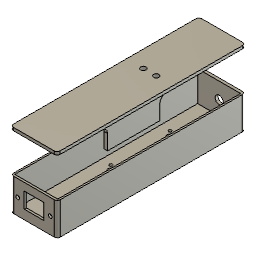
box_bridge_RS485_CAN v7 (Autodesk Fusion 360 design; units mm, degrees)
Autodesk Fusion 360 part; units mm, degrees
sketch "Sketch1" plane through (0, 0, 0) normal (0, 1, 0) x (1, 0, 0)
  line L0 (-27.5618, 41.4437) -> (-7.0618, 41.4437)
  line L1 (-7.0618, 41.4437) -> (-7.0618, -44.5563)
  line L2 (-7.0618, -44.5563) -> (-27.5618, -44.5563)
  line L3 (-27.5618, -44.5563) -> (-27.5618, 41.4437)
  line L4 (-17.3118, 41.4437) -> (-17.3118, -44.5563) construction
  line L5 (-7.0618, -1.5563) -> (-27.5618, -1.5563) construction
  line L6 (-7.0618, 24.2704) -> (-27.5618, 24.2704) construction
  line L7 (-17.3118, 24.2704) -> (-17.3118, -26.7296) construction
  circle A0 centre (-17.3118, 24.2704) radius 1.5
  circle A1 centre (-17.3118, -26.7296) radius 1.5
  dimension "d1" = 20.5
  dimension "d2" = 86
  dimension "d3" = 51
  dimension "d4" = 3
  dimension "d5" = 3
  constraint horizontal L0
  constraint vertical L1
  constraint horizontal L2
  constraint vertical L3
  constraint midpoint L0 L4.start
  constraint midpoint L2 L4.end
  constraint midpoint L1 L5.start
  constraint midpoint L3 L5.end
  constraint coincident L1 L6.start
  constraint coincident L3 L6.end
  constraint perpendicular L3 L6
  constraint midpoint L6 L7.start
  constraint perpendicular L6 L7
  constraint coincident L7.start A0.centre
  constraint coincident L7.end A1.centre
  measures "d1" distance of L0.start L0.end
  measures "d2" distance of L0.end L1.end
  measures "d3" distance of L7.start L7.end
  measures "d4" diameter of A0
  measures "d5" diameter of A1
extrude "Extrude1" add sketch "Sketch1" along normal blind 19.7 makes body 1
sketch "Sketch2" plane through (0, 19.7, 0) normal (0, 1, 0) x (-1, 0, 0)
  circle A0 centre (17.3118, -24.2704) radius 1.5
  circle A1 centre (17.3118, 26.7296) radius 1.5
  line L0 (27.5618, 44.5563) -> (7.0618, 44.5563)
  line L1 (7.0618, 44.5563) -> (7.0618, -41.4437)
  line L2 (7.0618, -41.4437) -> (27.5618, -41.4437)
  line L3 (27.5618, -41.4437) -> (27.5618, 44.5563)
extrude "Extrude2" cut sketch "Sketch2" against normal blind 5 bodies 1
sketch "Sketch3" plane through (0, 14.7, 0) normal (0, 1, 0) x (-1, 0, 0)
  circle A0 centre (17.3118, 26.7296) radius 1.5
  circle A1 centre (17.3118, -24.2704) radius 1.5
  line L0 (27.5618, -41.4437) -> (27.5618, 44.5563)
  line L1 (27.5618, 44.5563) -> (7.0618, 44.5563)
  line L2 (7.0618, 44.5563) -> (7.0618, -41.4437)
  line L3 (7.0618, -41.4437) -> (27.5618, -41.4437)
  line L4 (17.3118, 26.7296) -> (17.3118, 10.2296) construction
  line L5 (17.3118, 10.2296) -> (11.8118, 10.2296) construction
  line L6 (17.3118, 10.2296) -> (22.8118, 10.2296) construction
  circle A2 centre (22.8118, 10.2296) radius 1.75
  circle A3 centre (17.3118, 10.2296) radius 1.75
  circle A4 centre (11.8118, 10.2296) radius 1.75
  dimension "d10" = 16.5
  dimension "d11" = 5.5
  dimension "d12" = 5.5
  dimension "d13" = 3.5
  dimension "d14" = 3.5
  dimension "d15" = 3.5
  constraint coincident A0.centre L4.start
  constraint parallel L2 L4
  constraint perpendicular L4 L5
  constraint perpendicular L4 L6
  constraint coincident L6.end A2.centre
  constraint coincident L4.end L5.start
  constraint coincident L5.end A4.centre
  measures "d10" distance of A0.centre L4.end
  measures "d11" distance of L4.end L5.end
  measures "d12" distance of L4.end L6.end
  measures "d13" diameter of A2
  measures "d14" diameter of A3
  measures "d15" diameter of A4
extrude "Extrude3" add sketch "Sketch3" along normal blind 5 contours A2 | A3 | A4 bodies 1
sketch "Sketch4" plane through (0, 0, 0) normal (0, 0, 1) x (1, 0, 0)
  line L0 (0, 0) -> (40, 0)
  line L1 (40, 0) -> (40, 26)
  line L2 (40, 26) -> (0, 26)
  line L3 (0, 26) -> (0, 0)
  line L4 (0, 0) -> (40, 0) construction
  line L5 (40, 0) -> (40, 6) construction
  line L6 (40, 6) -> (0, 6) construction
  line L7 (0, 6) -> (0, 0) construction
  line L8 (20, 6) -> (20, 26) construction
  line L9 (20, 6) -> (28.5, 6) construction
  line L10 (28.5, 6) -> (28.5, 19.5) construction
  line L11 (28.5, 19.5) -> (20, 19.5) construction
  line L12 (20, 19.5) -> (20, 6) construction
  line L13 (20, 6) -> (11.5, 6) construction
  line L14 (11.5, 6) -> (11.5, 19.5) construction
  line L15 (11.5, 19.5) -> (20, 19.5) construction
  line L16 (20, 19.5) -> (20, 6) construction
  line L17 (0, 0) -> (40, 0) construction
  line L18 (40, 0) -> (40, 12) construction
  line L19 (40, 12) -> (0, 12) construction
  line L20 (0, 12) -> (0, 0) construction
  line L21 (59.0811, 36.4997) -> (20, 36.4997) construction
  line L22 (20, 36.4997) -> (20, 6) construction
  line L23 (20, 6) -> (59.0811, 6) construction
  line L24 (59.0811, 6) -> (59.0811, 36.4997) construction
  line L25 (20, 6) -> (34, 6) construction
  line L26 (34, 6) -> (34, 26) construction
  line L27 (34, 26) -> (20, 26) construction
  line L28 (20, 26) -> (20, 6) construction
  line L29 (20, 6) -> (6, 6) construction
  line L30 (6, 6) -> (6, 26) construction
  line L31 (6, 26) -> (20, 26) construction
  line L32 (20, 26) -> (20, 6) construction
  line L33 (11.5, 6) -> (28.5, 6)
  line L34 (28.5, 6) -> (28.5, 19.5)
  line L35 (28.5, 19.5) -> (11.5, 19.5)
  line L36 (11.5, 19.5) -> (11.5, 6)
  circle A0 centre (34, 12) radius 1.6
  circle A1 centre (6, 12) radius 1.6
  dimension "d18" = 40
  dimension "d19" = 26
  dimension "d20" = 6
  dimension "d21" = 8.5
  dimension "d22" = 13.5
  dimension "d23" = 8.5
  dimension "d24" = 12
  dimension "d25" = 14
  dimension "d26" = 14
  dimension "d27" = 3.2
  dimension "d28" = 3.2
  constraint horizontal L0
  constraint vertical L1
  constraint horizontal L2
  constraint vertical L3
  constraint coincident L0.start L3.end
  constraint horizontal L4
  constraint vertical L5
  constraint horizontal L6
  constraint vertical L7
  constraint midpoint L6 L8.start
  constraint midpoint L2 L8.end
  constraint perpendicular L2 L8
  constraint horizontal L9
  constraint vertical L10
  constraint horizontal L11
  constraint vertical L12
  constraint horizontal L13
  constraint vertical L14
  constraint horizontal L15
  constraint vertical L16
  constraint horizontal L17
  constraint vertical L18
  constraint horizontal L19
  constraint vertical L20
  constraint coincident L1 L18.end
  constraint horizontal L21
  constraint vertical L22
  constraint horizontal L23
  constraint vertical L24
  constraint horizontal L25
  constraint vertical L26
  constraint horizontal L27
  constraint vertical L28
  constraint horizontal L29
  constraint vertical L30
  constraint horizontal L31
  constraint vertical L32
  constraint horizontal L33
  constraint vertical L34
  constraint horizontal L35
  constraint vertical L36
  constraint coincident L19 A0.centre
  constraint coincident L26 A0.centre
  constraint coincident L19 A1.centre
  constraint coincident L30 A1.centre
  measures "d18" distance of L0.start L0.end
  measures "d19" distance of L0.start L2.end
  measures "d20" distance of L0.start L6.end
  measures "d21" distance of L8.start L9.end
  measures "d22" distance of L8.start L11.end
  measures "d23" distance of L8.start L13.end
  measures "d24" distance of L0.start L19.end
  measures "d25" distance of L8.start L25.end
  measures "d26" distance of L8.start L29.end
  measures "d27" diameter of A0
  measures "d28" diameter of A1
extrude "Extrude4" add sketch "Sketch4" along normal blind 1.9 separate body makes body 2
extrude "Extrude5" add 1 faces at (13.3333, 0, 0.6333) along direction (0, -1, 0) blind 2 on bodies 2 bodies 2
sketch "Sketch5" plane through (0, 0, 0) normal (0, 0, -1) x (-1, 0, 0)
  line L0 (-11.5, 19.5) -> (-11.5, 6)
  line L1 (-11.5, 6) -> (-28.5, 6)
  line L2 (-28.5, 6) -> (-28.5, 19.5)
  line L3 (-28.5, 19.5) -> (-11.5, 19.5)
  circle A0 centre (-34, 12) radius 1.6
  circle A1 centre (-6, 12) radius 1.6
  line L4 (0, -2) -> (0, 26)
  line L5 (0, 26) -> (-40, 26)
  line L6 (-40, 26) -> (-40, -2)
  line L7 (-40, -2) -> (0, -2)
  line L8 (-40, -2) -> (0, -2)
  line L9 (0, -2) -> (0, 0)
  line L10 (0, 0) -> (-40, 0)
  line L11 (-40, 0) -> (-40, -2)
  dimension "d33" = 2
  constraint horizontal L8
  constraint vertical L9
  constraint horizontal L10
  constraint vertical L11
  constraint coincident L6.end L7.start
  measures "d33" distance of L6.end L10.end
extrude "Extrude6" add sketch "Sketch5" along normal blind 160 contours L4 L6 L7 L8 L9 L10 L11 bodies 2
sketch "Sketch6" plane through (0, 0, 0) normal (0, 1, 0) x (-1, 0, 0)
  line L0 (0, 0) -> (-40, 0)
  line L1 (-40, 0) -> (-40, -160)
  line L2 (-40, -160) -> (0, -160)
  line L3 (0, -160) -> (0, 0)
  line L4 (-40, -160) -> (0, -160)
  line L5 (0, -160) -> (0, -157.5)
  line L6 (0, -157.5) -> (-40, -157.5)
  line L7 (-40, -157.5) -> (-40, -160)
  dimension "d36" = 2.5
  constraint horizontal L4
  constraint vertical L5
  constraint horizontal L6
  constraint vertical L7
  constraint coincident L1.end L2.start
  measures "d36" distance of L1.end L6.end
extrude "Extrude7" add sketch "Sketch6" along normal blind 26 contours L1 L2 L3 L4 L5 L6 L7 bodies 2
sketch "Sketch7" plane through (0, 0, -160) normal (0, 0, -1) x (-1, 0, 0)
  line L0 (-40, 26) -> (-40, -2)
  line L1 (-40, -2) -> (0, -2)
  line L2 (0, -2) -> (0, 26)
  line L3 (0, 26) -> (-40, 26)
  line L4 (-20, 26) -> (-20, -2) construction
  line L5 (0, 12) -> (-40, 12) construction
  circle A0 centre (-20, 12) radius 3.5
  dimension "d39" = 7
  constraint midpoint L3 L4.start
  constraint midpoint L1 L4.end
  constraint midpoint L2 L5.start
  constraint midpoint L0 L5.end
  constraint midpoint L4 A0.centre
  measures "d39" diameter of A0
extrude "Extrude8" cut sketch "Sketch7" against normal blind 3 contours A0 bodies 2
move_body "Move1" bodies 1 to x (1, 0, 0) y (0, 1, 0) z (0, 0, 1) at (37.1076, 0, -91.1851)
sketch "Sketch8" plane through (0, 0, 0) normal (0, 1, 0) x (-1, 0, 0)
  line L0 (-40, -157.5) -> (0, -157.5)
  line L1 (0, -157.5) -> (0, 0)
  line L2 (0, 0) -> (-40, 0)
  line L3 (-40, 0) -> (-40, -157.5)
  line L4 (-40, -64.3303) -> (0, -64.3303) construction
  line L5 (0, -64.3303) -> (0, -115.3303) construction
  line L6 (0, -115.3303) -> (-40, -115.3303) construction
  line L7 (-40, -115.3303) -> (-40, -64.3303) construction
  line L8 (-20, 0) -> (-20, -157.5) construction
  circle A0 centre (-20, -64.3303) radius 2.5
  circle A1 centre (-20, -115.3303) radius 2.5
  dimension "d42" = 51
  dimension "d43" = 5
  dimension "d44" = 5
  constraint horizontal L4
  constraint vertical L5
  constraint horizontal L6
  constraint vertical L7
  constraint coincident L1 L5.end
  constraint coincident L3 L4.start
  constraint midpoint L2 L8.start
  constraint midpoint L0 L8.end
  constraint midpoint L4 A0.centre
  constraint midpoint L6 A1.centre
  measures "d42" distance of L4.start L6.end
  measures "d43" diameter of A0
  measures "d44" diameter of A1
extrude "Extrude9" add sketch "Sketch8" along normal blind 6 contours A0 | A1 bodies 2
sketch "Sketch9" plane through (0, 6, 0) normal (0, 1, 0) x (-1, 0, 0)
  circle A0 centre (-20, -64.3303) radius 2.5
  circle A1 centre (-20, -64.3303) radius 1.25
  dimension "d47" = -1.25
sketch "Sketch10" plane through (0, 6, 0) normal (0, 1, 0) x (-1, 0, 0)
  circle A0 centre (-20, -115.3303) radius 2.5
  circle A1 centre (-20, -115.3303) radius 1.25
  dimension "d48" = -1.25
extrude "Extrude10" add sketch "Sketch10" along normal blind 4 contours A1 bodies 2
extrude "Extrude11" add sketch "Sketch9" along normal blind 4 contours A1 bodies 2
sketch "Sketch11" plane through (0, 0, 0) normal (0, 1, 0) x (-1, 0, 0)
  circle A0 centre (-20, -64.3303) radius 2.5
  circle A1 centre (-20, -115.3303) radius 2.5
  line L0 (-40, -157.5) -> (0, -157.5)
  line L1 (0, -157.5) -> (0, 0)
  line L2 (0, 0) -> (-40, 0)
  line L3 (-40, 0) -> (-40, -157.5)
  line L4 (-40, 0) -> (-38.5, 0)
  line L5 (-38.5, 0) -> (-38.5, -157.5)
  line L6 (-38.5, -157.5) -> (-40, -157.5)
  line L7 (-40, -157.5) -> (-40, 0)
  line L8 (0, 0) -> (-1.5, 0)
  line L9 (-1.5, 0) -> (-1.5, -157.5)
  line L10 (-1.5, -157.5) -> (0, -157.5)
  line L11 (0, -157.5) -> (0, 0)
  dimension "d53" = 1.5
  dimension "d54" = 1.5
  constraint horizontal L4
  constraint vertical L5
  constraint horizontal L6
  constraint vertical L7
  constraint coincident L2.end L3.start
  constraint horizontal L8
  constraint vertical L9
  constraint horizontal L10
  constraint vertical L11
  constraint coincident L1.end L2.start
  measures "d53" distance of L2.end L4.end
  measures "d54" distance of L1.end L8.end
extrude "Extrude12" add sketch "Sketch11" along normal blind 26 contours L0 L2 L3 L4 L5 L6 L7 | L0 L1 L2 L8 L9 L10 L11 bodies 2
fillet "Fillet1" radius 2.5 4 edges at (0, 12, -160) (0, 12, 1.9) (40, 12, -160) (40, 12, 1.9) on bodies 2
sketch "Sketch12" plane through (0, 0, 0) normal (0, 1, 0) x (-1, 0, 0)
  circle A0 centre (-20, -115.3303) radius 2.5
  circle A1 centre (-20, -64.3303) radius 2.5
  line L0 (-38.5, 0) -> (-38.5, -157.5)
  line L1 (-38.5, -157.5) -> (-1.5, -157.5)
  line L2 (-1.5, -157.5) -> (-1.5, 0)
  line L3 (-1.5, 0) -> (-38.5, 0)
  line L4 (-20, -112.8303) -> (-1.5, -112.8303) construction
  line L5 (-1.5, -112.8303) -> (-1.5, -97.8303) construction
  line L6 (-1.5, -97.8303) -> (-20, -97.8303) construction
  line L7 (-20, -97.8303) -> (-20, -112.8303) construction
  line L8 (-20, -112.8303) -> (-38.5, -112.8303) construction
  line L9 (-38.5, -112.8303) -> (-38.5, -97.8303) construction
  line L10 (-38.5, -97.8303) -> (-20, -97.8303) construction
  line L11 (-20, -97.8303) -> (-20, -112.8303) construction
  line L12 (-20, -97.8303) -> (-14.5, -97.8303) construction
  line L13 (-14.5, -97.8303) -> (-14.5, -112.8303) construction
  line L14 (-14.5, -112.8303) -> (-20, -112.8303) construction
  line L15 (-20, -112.8303) -> (-20, -97.8303) construction
  line L16 (-20, -112.8303) -> (-25.5, -112.8303) construction
  line L17 (-25.5, -112.8303) -> (-25.5, -97.8303) construction
  line L18 (-25.5, -97.8303) -> (-20, -97.8303) construction
  line L19 (-20, -97.8303) -> (-20, -112.8303) construction
  circle A2 centre (-14.5, -97.8303) radius 2.25
  circle A3 centre (-25.5, -97.8303) radius 2.25
  dimension "d59" = 15
  dimension "d60" = 15
  dimension "d61" = 5.5
  dimension "d62" = 5.5
  dimension "d63" = 4.5
  dimension "d64" = 4.5
  constraint horizontal L4
  constraint vertical L5
  constraint horizontal L6
  constraint vertical L7
  constraint coincident A0 L4.start
  constraint horizontal L8
  constraint vertical L9
  constraint horizontal L10
  constraint vertical L11
  constraint horizontal L12
  constraint vertical L13
  constraint horizontal L14
  constraint vertical L15
  constraint horizontal L16
  constraint vertical L17
  constraint horizontal L18
  constraint vertical L19
  constraint coincident L12.end L13.start
  constraint coincident L17.end L18.start
  measures "d59" distance of L4.start L6.end
  measures "d60" distance of L4.start L6.end
  measures "d61" distance of L6.end L12.end
  measures "d62" distance of L4.start L16.end
  measures "d63" diameter of A2
  measures "d64" diameter of A3
extrude "Extrude13" add sketch "Sketch12" along normal blind 47.1 separate body contours A2 | A3 makes body 3 at (27.5733, 31.4, -98.7043) makes body 4 at (16.5733, 31.4, -98.7043)
ref_plane "WorkPlane1" through (0, 37, 0) normal (0, 1, 0) x (0, 0, 1)
sketch "Sketch13" plane through (0, 37, 0) normal (0, 1, 0) x (1, 0, 0)
  line L0 (40.0982, -2.0564) -> (-0.1172, -2.0564)
  line L1 (-0.1172, -2.0564) -> (-0.1172, 160.1441)
  line L2 (-0.1172, 160.1441) -> (40.0982, 160.1441)
  line L3 (40.0982, 160.1441) -> (40.0982, -2.0564)
  constraint horizontal L0
  constraint vertical L1
  constraint horizontal L2
  constraint vertical L3
extrude "Extrude14" add sketch "Sketch13" along normal blind 2 separate body makes body 5
extrude "Extrude15" add 1 faces at (26.6931, 39, -52.0104) along direction (0, 1, 0) blind 2 on bodies 5 bodies 5
move_body "Move2" bodies 5 to x (1, 0, 0) y (0, 1, 0) z (0, 0, 1) at (0, -12.4, 0)
fillet "Fillet2" radius 2.5 4 edges at (-0.1172, 26.6, -160.1441) (40.0982, 26.6, -160.1441) (-0.1172, 26.6, 2.0564) (40.0982, 26.6, 2.0564) on bodies 5
combine "Combine1" operation cut target body 5 tool bodies 2 keep tools
move_body "Move3" bodies 5 to x (1, 0, 0) y (0, 1, 0) z (0, 0, 1) at (0, 37.7, 0)
extrude "Extrude16" cut 1 faces at (14.1604, 62.3, 2.0043) along direction (0, 1, 0) blind 1.4 on bodies 5 bodies 5
move_body "Move4" bodies 5 to x (1, 0, 0) y (0, 1, 0) z (0, 0, 1) at (0, -33.4, 0)
combine "Combine2" operation cut target body 5 tool bodies 4 3 keep tools
move_body "Move5" bodies 5 to x (1, 0, 0) y (0, 1, 0) z (0, 0, 1) at (0, 29.6, 0)
sketch "Sketch14" plane through (0, 58.5, 0) normal (0, -1, 0) x (1, 0, 0)
  circle A0 centre (25.5, -97.8303) radius 2.25
  circle A1 centre (14.5, -97.8303) radius 2.25
  line L0 (38.5, -157.5) -> (38.5, 0)
  line L1 (38.5, 0) -> (1.5, 0)
  line L2 (1.5, 0) -> (1.5, -157.5)
  line L3 (1.5, -157.5) -> (38.5, -157.5)
  line L4 (38.5, -87.9718) -> (35.5, -87.9718)
  line L5 (35.5, -87.9718) -> (35.5, -42.9718)
  line L6 (35.5, -42.9718) -> (38.5, -42.9718)
  line L7 (38.5, -42.9718) -> (38.5, -87.9718)
  line L8 (35.5, -87.9718) -> (1.5, -87.9718) construction
  line L9 (35.5, -42.9718) -> (1.5, -42.9718) construction
  line L10 (1.5, -87.9718) -> (4.5, -87.9718)
  line L11 (4.5, -87.9718) -> (4.5, -42.9718)
  line L12 (4.5, -42.9718) -> (1.5, -42.9718)
  line L13 (1.5, -42.9718) -> (1.5, -87.9718)
  dimension "d76" = 3
  dimension "d77" = 45
  dimension "d78" = 3
  constraint horizontal L4
  constraint vertical L5
  constraint horizontal L6
  constraint vertical L7
  constraint coincident L0 L4.start
  constraint coincident L2 L8.end
  constraint perpendicular L2 L8
  constraint coincident L2 L9.end
  constraint perpendicular L2 L9
  constraint horizontal L10
  constraint vertical L11
  constraint horizontal L12
  constraint vertical L13
  constraint coincident L9 L11.end
  measures "d76" distance of L4.start L4.end
  measures "d77" distance of L4.start L6.end
  measures "d78" distance of L8.end L10.end
extrude "Extrude17" add sketch "Sketch14" along normal blind 18 contours L0 L4 L5 L6 L7 | L2 L10 L11 L12 L13 bodies 5
fillet "Fillet3" radius 5 6 edges at (37, 58.5, -87.9718) (35.5, 58.5, -65.4718) (3, 58.5, -87.9718) (4.5, 58.5, -65.4718) (3, 58.5, -42.9718) (37, 58.5, -42.9718) on bodies 5
fillet "Fillet4" radius 1.5 4 edges at (1.5, 59.2, 0) (38.5, 59.2, 0) (38.5, 59.2, -157.5) (1.5, 59.2, -157.5) on bodies 5
hidden bodies 1 3 4
equation "d21 = ( 17 / 2 ) * 1 mm"
equation "d23 = ( 17 / 2 ) * 1 mm"
